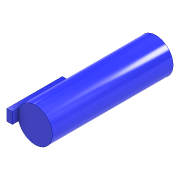
# Autodesk Inventor part: LiPo_Akku_18650_Dummy
Saved by Autodesk Inventor 2020 (Build 240168000, 168)
## iProperties
Created: 2020-08-23
Part Number: LiPo_Akku_18650_Dummy
Material: Generisch
Document SubType Name: Modeling
Designer: uhlma
Density: 1 g/cm^3
Appearance: Blau - Wandfarbe - glänzend
Author: uhlma
Autodesk Inventor part; units mm, degrees
ref_plane "XZ Plane" through (0, 0, 0) normal (0, 1, 0) x (-1, 0, 0)
ref_plane "XY Plane" through (0, 0, 0) normal (0, 0, 1) x (1, 0, 0)
sketch "Skizze1" plane through (0, 0, 0) normal (0, 0, 1) x (1, 0, 0)
  circle A0 centre (0, 0) radius 9.3
  dimension "d0" = 18.6
  constraints: 1 centre point, 1 coincident
  measures "d0" diameter of A0
extrude "Extrusion1" add sketch "Skizze1" along normal mid plane 65.2
ref_plane "Arbeitsebene1" through (-9.3, 0, 0) normal (1, 0, 0) x (0, 1, 0)
sketch "Skizze2" plane through (-9.3, 0, 0) normal (1, 0, 0) x (0, 1, 0)
  line L0 (3, 35.6) -> (-3, 35.6)
  line L1 (-3, 35.6) -> (-3, 5.6)
  line L2 (-3, 5.6) -> (3, 5.6)
  line L3 (3, 5.6) -> (3, 35.6)
  line L4 (9.3, 32.6) -> (-9.3, 32.6) projected
  point P0 (0, 0)
  point P1 (0, 5.6)
  dimension "d3" = 6
  dimension "d4" = 30
  dimension "d5" = 27
  constraints: 8 end point, 2 parallel, 1 horizontal, 1 midpoint, 1 perpendicular, 1 vertical alignment
  measures "d3" distance of L0.start L0.end
  measures "d4" distance of L2.end L0.start
  measures "d5" distance between parallel lines of L4 L2
extrude "Extrusion2" add sketch "Skizze2" against normal blind 3
